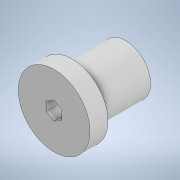
# Autodesk Inventor part: Hex Adapter
Saved by Autodesk Inventor 2020 (Build 240168000, 168)
## iProperties
Created: 2020-01-26
Part Number: Hex Adapter
Material: Generic
Document SubType Name: Modeling
Designer: autum
Density: 1 g/cm^3
Appearance: Default
Author: autum
Autodesk Inventor part; units mm, degrees
ref_plane "YZ Plane" through (0, 0, 0) normal (1, 0, 0) x (0, 1, 0)
ref_plane "XZ Plane" through (0, 0, 0) normal (0, 1, 0) x (-1, 0, 0)
ref_plane "XY Plane" through (0, 0, 0) normal (0, 0, 1) x (1, 0, 0)
sketch "Sketch1" plane through (0, 0, 0) normal (0, 0, 1) x (1, 0, 0)
  circle A0 centre (0, 0) radius 17.526
  dimension "d0" = 35.052
  constraints: 1 centre point, 1 coincident
  measures "d0" diameter of A0
extrude "Extrusion1" add sketch "Sketch1" along normal blind 38.1
sketch "Sketch2" plane through (0, 0, 38.1) normal (0, 0, 1) x (1, 0, 0)
  circle A0 centre (0, 0) radius 25.4
  dimension "d3" = 50.8
  constraints: 1 centre point
  measures "d3" diameter of A0
extrude "Extrusion2" add sketch "Sketch2" along normal blind 12.7
sketch "Sketch3" plane through (0, 0, 50.8) normal (0, 0, 1) x (1, 0, 0)
  line L0 (0, -6.35) -> (-5.4993, -3.175)
  line L1 (-5.4993, -3.175) -> (-5.4993, 3.175)
  line L2 (-5.4993, 3.175) -> (0, 6.35)
  line L3 (0, 6.35) -> (5.4993, 3.175)
  line L4 (5.4993, 3.175) -> (5.4993, -3.175)
  line L5 (5.4993, -3.175) -> (0, -6.35)
  point P0 (0, 0)
  point P1 (0, 0)
  dimension "d7" = 12.7
  constraints: 12 end point, 1 coincident, 13 other
  measures "d7" distance of L0.start L2.end
extrude "Extrusion3" cut sketch "Sketch3" against normal through all
body "Solid1"
